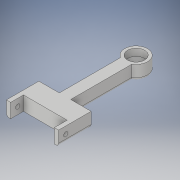
# Autodesk Inventor part: Tarea 16 P2
Saved by Autodesk Inventor 2019 (Build 230136000, 136)
## iProperties
Created: 2020-02-28
Part Number: Tarea 16 P2
Material: Generic
Document SubType Name: Modeling
Designer: juanc
Density: 1 g/cm^3
Appearance: Default
Author: juanc
Autodesk Inventor part; units mm, degrees
ref_plane "YZ Plane" through (0, 0, 0) normal (1, 0, 0) x (0, 1, 0)
ref_plane "XZ Plane" through (0, 0, 0) normal (0, 1, 0) x (-1, 0, 0)
ref_plane "XY Plane" through (0, 0, 0) normal (0, 0, 1) x (1, 0, 0)
sketch "Sketch1" plane through (0, 0, 0) normal (0, 1, 0) x (-1, 0, 0)
  line L0 (3, -9.02) -> (33.75, -9.02)
  line L1 (33.75, -9.02) -> (33.75, 0)
  line L2 (33.75, 0) -> (36.75, 0)
  line L3 (36.75, 0) -> (36.75, -22.86)
  line L4 (36.75, -22.86) -> (22.375, -22.86)
  line L5 (22.375, -22.86) -> (22.375, -65.9087)
  line L6 (14.375, -22.86) -> (14.375, -65.9087)
  line L7 (18.375, -22.86) -> (18.375, -72.86) construction
  arc A0 (14.375, -65.9087) -> (22.375, -65.9087) centre (18.375, -72.86) ccw
  line L8 (3, -9.02) -> (3, 0)
  line L9 (3, 0) -> (0, 0)
  line L10 (0, 0) -> (0, -22.86)
  line L11 (14.375, -22.86) -> (0, -22.86)
  dimension "d2" = 30.75
  dimension "d3" = 3
  dimension "d4" = 22.86
  dimension "d9" = 8
  dimension "d12" = 4
  dimension "d13" = 8.02
  dimension "d15" = 14.375
  dimension "d16" = 3
  dimension "d17" = 22.86
  constraints: 24 end point, 6 perpendicular, 3 vertical, 2 horizontal, 2 point on circle, 1 centre point, 1 coincident, 1 parallel, 1 point on line
  measures "d2" distance of L0.start L0.end
  measures "d3" distance of L1.end L2.end
  measures "d4" distance of L2.end L3.end
  measures "d9" distance between parallel lines of L5 L6
  measures "d12" distance between parallel lines of L7 L5
  measures "d13" radius of A0
  measures "d15" distance of L6.start L10.end
  measures "d16" distance of L8.end L9.end
  measures "d17" distance of L9.end L10.end
extrude "Extrusion1" add sketch "Sketch1" along normal blind 10
sketch "Sketch2" plane through (0, 0, 0) normal (1, 0, 0) x (0, 0, -1)
  circle A0 centre (5, 5) radius 1.5
  line L0 (0, 0) -> (0, 10) projected
  line L1 (0, 10) -> (22.86, 10) projected
  dimension "d23" = 5
  dimension "d24" = 5
  dimension "d25" = 3
  constraints: 1 centre point
  measures "d23" distance from line of L1 A0.centre
  measures "d24" distance from line of L0 A0.centre
  measures "d25" diameter of A0
extrude "Extrusion2" cut sketch "Sketch2" against normal blind 3
sketch "Sketch3" plane through (-36.75, 0, -22.86) normal (-1, 0, 0) x (0, 0, 1)
  circle A0 centre (17.86, 5) radius 1.5 projected
  circle A1 centre (17.86, 5) radius 1.5
  point P0 (22.86, 0)
  constraints: 1 centre point, 1 coincident
extrude "Extrusion3" cut sketch "Sketch3" against normal blind 3
sketch "Sketch4" plane through (0, 10, 0) normal (0, 1, 0) x (1, 0, 0)
  arc A0 (-14.375, 65.9087) -> (-22.375, 65.9087) centre (-18.375, 72.86) ccw projected
  circle A1 centre (-18.375, 72.86) radius 6.015
  point P0 (0, 0)
  dimension "d30" = 12.03
  constraints: 1 centre point, 1 coincident
  measures "d30" diameter of A1
extrude "Extrusion4" cut sketch "Sketch4" against normal blind 5
fillet "Fillet1" radius 2 7 edges at (-18.375, 0, -80.88) (-14.375, 0, -44.3844) (-7.1875, 0, -22.86) (-29.5625, 0, -22.86) (0, 0, -11.43) (-36.75, 0, -11.43) (-22.375, 0, -44.3844)
body "Solid1"
